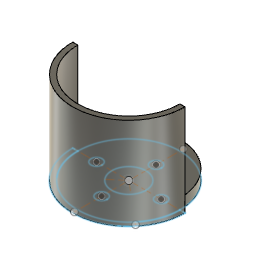
motor-case (Autodesk Fusion 360 design; units mm, degrees)
Autodesk Fusion 360 part; units mm, degrees
sketch "Sketch1" plane through (0, 0, 0) normal (0, 0, 1) x (1, 0, 0)
  line L0 (50, 55) -> (66, 55) construction
  line L1 (50, 55) -> (34, 55) construction
  line L2 (50, 55) -> (50, 39) construction
  line L3 (50, 55) -> (50, 71) construction
  circle A0 centre (40.5, 55) radius 1.6
  circle A1 centre (50, 63) radius 1.6
  circle A2 centre (59.5, 55) radius 1.6
  circle A3 centre (50, 47) radius 1.6
  line L4 (65, 55) -> (66, 55)
  line L5 (35, 55) -> (34, 55)
  line L6 (50, 55) -> (46.1698, 51.7861) construction
  arc A4 (61.4907, 45.3582) -> (65, 55) centre (50, 55) ccw
  arc A5 (35, 55) -> (38.5093, 45.3582) centre (50, 55) ccw
  circle A6 centre (50, 55) radius 5
  line L7 (34, 55) -> (33.5, 55)
  line L8 (66, 55) -> (66.5, 55)
  circle A7 centre (50, 55) radius 15
  line L9 (50, 55) -> (53.8302, 51.7861) construction
  line L10 (61.4907, 45.3582) -> (62.2567, 44.7154) construction
  arc A8 (33.5, 55) -> (66.5, 55) centre (50, 55) ccw
  point P0 (59.5, 55)
  point P1 (50, 63)
  point P2 (50, 47)
  point P3 (40.5, 55)
  dimension "d23" = 30
  dimension "d25" = 8
  dimension "d26" = 8
  dimension "d27" = 9.5
  dimension "d28" = 9.5
  dimension "d29" = 3.2
  dimension "d30" = 3.2
  dimension "d31" = 3.2
  dimension "d32" = 3.2
  dimension "d33" = 140
  dimension "d34" = 80
  dimension "d41" = 10
  dimension "d44" = 33
  constraint coincident L0.start L1.start
  constraint horizontal L0
  constraint parallel L0 L1
  constraint perpendicular L1 L2
  constraint parallel L2 L3
  constraint coincident L0 P0
  constraint coincident L3 P1
  constraint coincident L2 P2
  constraint coincident L1 P3
  constraint coincident P3 A0.centre
  constraint coincident P1 A1.centre
  constraint coincident P0 A2.centre
  constraint coincident P2 A3.centre
  constraint coincident L0 L4.start
  constraint coincident L5.start A4
  constraint coincident L1 L5.start
  constraint coincident A4.start L9
  constraint concentric A4 A5
  constraint concentric A5 A6
  constraint parallel L1 L7
  constraint parallel L0 L8
  constraint coincident A5.end A7
  constraint coincident A6 L9.end
  constraint collinear L9 L10
  constraint coincident A6 L6.end
  measures "d23" diameter of A4
  measures "d25" distance of L0.start A1.centre
  measures "d26" distance of L0.start P2
  measures "d27" distance of L0.start P0
  measures "d28" distance of L0.start P3
  measures "d29" diameter of A0
  measures "d30" diameter of A1
  measures "d31" diameter of A2
  measures "d32" diameter of A3
  measures "d33" angle of L5 L6
  measures "d34" angle of L6 L9
  measures "d41" diameter of A6
  measures "d44" diameter of A8
extrude "Extrude7" add sketch "Sketch1" along normal blind 3 contours A4 A5 A7
extrude "Extrude8" add sketch "Sketch1" along normal blind 27 contours L4 L5 A4 A5 L7 L8 A7 A8
chamfer "Chamfer2" distance 0.5 distance2 2 1 edges at (45.3384, 56.8081, 3) measured on face at (42.065, 60.0544, 3)
chamfer "Chamfer3" distance 2 distance2 1 4 edges at (58.0083, 55.5786, 0) (48.5083, 47.5786, 0) (39.0083, 55.5786, 0) (48.5083, 63.5786, 0) measured on face at (60.434, 56.2991, 2) measured on face at (50.934, 48.2991, 2) measured on face at (41.434, 56.2991, 2) measured on face at (51.0587, 64.1997, 2)
fillet "Fillet1" radius 1.5 2 edges at (65, 55, 1.5) (35, 55, 1.5)
sketch "Sketch2" plane through (0, 0, 0) normal (0, 1, 0) x (1, 0, 0)
named bodies: "motor-case"
